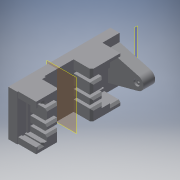
# Autodesk Inventor part: Assembly-jig-base
Saved by Autodesk Inventor 2018 (Build 220112000, 112)
## iProperties
Created: 2017-11-08
Part Number: Assembly-jig-base
Material: Generic
Document SubType Name: Modeling
Designer: xl0
Density: 1 g/cm^3
Appearance: Default
Author: xl0
Autodesk Inventor part; units mm, degrees
ref_plane "YZ Plane" through (0, 0, 0) normal (1, 0, 0) x (0, 1, 0)
ref_plane "XZ Plane" through (0, 0, 0) normal (0, 1, 0) x (-1, 0, 0)
ref_plane "Work Plane3" through (-2, 0, -40) normal (-1, 0, 0) x (0, 0, 1)
sketch "Sketch3" plane through (-2, 0, -8) normal (-1, 0, 0) x (0, -1, 0)
  line L0 (54.7526, 13.2) -> (67.7526, 13.2)
  line L1 (67.7526, 13.2) -> (67.7526, 3.2)
  line L2 (67.7526, 3.2) -> (54.7526, 3.2)
  line L3 (54.7526, 3.2) -> (54.7526, 13.2)
  line L4 (104.2526, 13.2) -> (117.2526, 13.2)
  line L5 (117.2526, 13.2) -> (117.2526, 3.2)
  line L6 (117.2526, 3.2) -> (104.2526, 3.2)
  line L7 (104.2526, 3.2) -> (104.2526, 13.2)
  line L8 (54.7526, -25.2) -> (67.7526, -25.2)
  line L9 (67.7526, -25.2) -> (67.7526, -35.2)
  line L10 (67.7526, -35.2) -> (54.7526, -35.2)
  line L11 (54.7526, -35.2) -> (54.7526, -25.2)
  line L12 (104.2526, -25.2) -> (117.2526, -25.2)
  line L13 (117.2526, -25.2) -> (117.2526, -35.2)
  line L14 (117.2526, -35.2) -> (104.2526, -35.2)
  line L15 (104.2526, -35.2) -> (104.2526, -25.2)
  line L16 (41.7526, -32) -> (41.7526, 8) projected
  line L17 (125.2526, 8) -> (125.2526, -32) projected
  line L18 (63.2526, 0) -> (63.2526, 3) projected
  line L19 (67.7526, 0) -> (67.7526, 3) projected
  line L20 (99.2526, 0) -> (99.2526, 3) projected
  line L21 (103.7526, 0) -> (103.7526, 3) projected
  line L22 (44.7526, 3) -> (122.2526, 3) projected
  line L23 (122.2526, -25) -> (44.7526, -25) projected
  line L24 (54.7526, -0.2) -> (67.7526, -0.2)
  line L25 (67.7526, -0.2) -> (67.7526, -11.8)
  line L26 (67.7526, -11.8) -> (54.7526, -11.8)
  line L27 (54.7526, -11.8) -> (54.7526, -0.2)
  line L28 (54.7526, -15.2) -> (67.7526, -15.2)
  line L29 (67.7526, -15.2) -> (67.7526, -21.8)
  line L30 (67.7526, -21.8) -> (54.7526, -21.8)
  line L31 (54.7526, -21.8) -> (54.7526, -15.2)
  line L32 (104.2526, -0.2) -> (117.2526, -0.2)
  line L33 (117.2526, -0.2) -> (117.2526, -11.8)
  line L34 (117.2526, -11.8) -> (104.2526, -11.8)
  line L35 (104.2526, -11.8) -> (104.2526, -0.2)
  line L36 (104.2526, -15.2) -> (117.2526, -15.2)
  line L37 (117.2526, -15.2) -> (117.2526, -21.8)
  line L38 (117.2526, -21.8) -> (104.2526, -21.8)
  line L39 (104.2526, -21.8) -> (104.2526, -15.2)
  line L40 (44.7526, 0) -> (122.2526, 0) projected
  line L41 (44.7526, -12) -> (122.2526, -12) projected
  line L42 (44.7526, -15) -> (122.2526, -15) projected
  line L43 (44.7526, -22) -> (122.2526, -22) projected
  line L44 (122.2526, 8) -> (122.2526, -32) projected
  line L45 (44.7526, -32) -> (44.7526, 8) projected
  line L46 (125.2526, 8) -> (122.2526, 8) projected
  line L47 (125.2526, -32) -> (122.2526, -32) projected
  dimension "d7" = 10
  dimension "d9" = 0.2
  dimension "d10" = 0.2
  dimension "d11" = 0.2
  dimension "d12" = 0.2
  dimension "d13" = 0.2
  dimension "d34" = 5
  dimension "d36" = 13
  dimension "d48" = 0.2
  dimension "d80" = 10
  constraints: 64 end point, 15 collinear, 15 parallel, 8 horizontal, 8 perpendicular, 4 equal length, 3 point on line
  measures "d7" distance of L0.end L1.end
  measures "d9" distance between parallel lines of L23 L8
  measures "d10" distance between parallel lines of L26 L41
  measures "d11" distance between parallel lines of L40 L24
  measures "d12" distance between parallel lines of L42 L28
  measures "d13" distance between parallel lines of L43 L30
  measures "d34" distance between parallel lines of L37 L44
  measures "d36" distance of L9.end L10.end
  measures "d48" distance between parallel lines of L22 L2
  measures "d80" distance between parallel lines of L11 L45
extrude "Extrusion2" add sketch "Sketch3" against normal blind 20 contours L0 L1 L2 L3 | L4 L5 L6 L7 | L8 L9 L10 L11 | L12 L13 L14 L15 | L24 L25 L26 L27 | L28 L29 L30 L31 | L32 L33 L34 L35 | L36 L37 L38 L39
sketch "Sketch10" plane through (-2, 0, -8) normal (-1, 0, 0) x (0, 0, 1)
  line L0 (13.2, -117.2526) -> (13.2, -129.2526)
  line L1 (13.2, -129.2526) -> (6.7, -129.2526)
  line L2 (6.7, -129.2526) -> (6.7, -125.4526)
  line L3 (6.7, -125.4526) -> (8.2, -125.4526)
  line L4 (6.7, -117.2526) -> (13.2, -117.2526)
  line L5 (8, -125.2526) -> (-32, -125.2526) projected
  line L6 (8, -125.2526) -> (8, -122.2526) projected
  line L7 (-32, -122.2526) -> (8, -122.2526) projected
  line L8 (-32, -125.2526) -> (-32, -122.2526) projected
  line L9 (13.2, -104.2526) -> (13.2, -117.2526) projected
  line L10 (-30.7, -129.2526) -> (-37.2, -129.2526)
  line L11 (-37.2, -129.2526) -> (-37.2, -104.2526)
  line L12 (-32.2, -125.4526) -> (-30.7, -125.4526)
  line L13 (-30.7, -125.4526) -> (-30.7, -129.2526)
  line L14 (-32.2, -125.4526) -> (-32.2, -122.0526)
  line L15 (-32.2, -122.0526) -> (-30.7, -122.0526)
  line L16 (-30.7, -122.0526) -> (-30.7, -117.2526)
  line L17 (8.2, -125.4526) -> (8.2, -122.0526)
  line L18 (8.2, -122.0526) -> (6.7, -122.0526)
  line L19 (6.7, -122.0526) -> (6.7, -117.2526)
  line L20 (13.2, -117.2526) -> (3.2, -117.2526) projected
  line L21 (-25.2, -104.2526) -> (-25.2, -117.2526) projected
  line L22 (-25.2, -117.2526) -> (-35.2, -117.2526) projected
  line L23 (-35.2, -117.2526) -> (-35.2, -104.2526) projected
  line L24 (-35.2, -104.2526) -> (-25.2, -104.2526) projected
  line L25 (-35.2, -117.2526) -> (-35.2, -104.2526) projected
  line L26 (-35.2, -104.2526) -> (-37.2, -104.2526)
  line L27 (13.2, -35.7526) -> (13.2, -54.7526)
  line L28 (5.2, -45.2526) -> (8.2, -45.2526)
  line L29 (8.2, -45.2526) -> (8.2, -35.7526)
  line L30 (8.2, -35.7526) -> (13.2, -35.7526)
  line L31 (-29.2, -45.2526) -> (-29.2, -54.7526)
  line L32 (-37.2, -67.7526) -> (-37.2, -35.7526)
  line L33 (-37.2, -35.7526) -> (-32.2, -35.7526)
  line L34 (-32.2, -35.7526) -> (-32.2, -45.2526)
  line L35 (-32.2, -45.2526) -> (-29.2, -45.2526)
  line L36 (8, -44.7526) -> (-32, -44.7526) projected
  line L37 (8, -44.7526) -> (8, -41.7526) projected
  line L38 (-32, -41.7526) -> (8, -41.7526) projected
  line L39 (-32, -44.7526) -> (-32, -41.7526) projected
  line L40 (13.2, -54.7526) -> (13.2, -67.7526) projected
  line L41 (13.2, -67.7526) -> (3.2, -67.7526) projected
  line L42 (3.2, -67.7526) -> (3.2, -54.7526) projected
  line L43 (3.2, -54.7526) -> (13.2, -54.7526) projected
  line L44 (3.2, -54.7526) -> (13.2, -54.7526) projected
  line L45 (-25.2, -54.7526) -> (-25.2, -67.7526) projected
  line L46 (-25.2, -67.7526) -> (-35.2, -67.7526) projected
  line L47 (-35.2, -67.7526) -> (-35.2, -54.7526) projected
  line L48 (-35.2, -54.7526) -> (-25.2, -54.7526) projected
  line L49 (-37.2, -67.7526) -> (-35.2, -67.7526)
  line L50 (5.2, -45.2526) -> (5.2, -54.7526)
  line L51 (-35.2, -54.7526) -> (-25.2, -54.7526) projected
  point P0 (8, 0)
  dimension "d50" = 0.2
  dimension "d54" = 12
  dimension "d58" = 0.2
  dimension "d59" = 0.2
  dimension "d60" = 1.5
  dimension "d61" = 0.2
  dimension "d71" = 0.5
  dimension "d72" = 0.2
  dimension "d75" = 6
  dimension "d77" = 5
  dimension "d78" = 0.2
  dimension "d79" = 0.5
  dimension "d83" = 3
  constraints: 54 end point, 12 collinear, 12 perpendicular, 5 horizontal, 4 point on line, 4 vertical, 3 parallel
  measures "d50" distance between parallel lines of L3 L5
  measures "d54" distance of L0.start L0.end
  measures "d58" distance between parallel lines of L17 L6
  measures "d59" distance between parallel lines of L18 L7
  measures "d60" distance of L17.end L18.end
  measures "d61" distance between parallel lines of L8 L14
  measures "d71" distance between parallel lines of L28 L36
  measures "d72" distance between parallel lines of L29 L37
  measures "d75" distance between parallel lines of L38 L30
  measures "d77" distance of L29.end L27.start
  measures "d78" distance between parallel lines of L39 L34
  measures "d79" distance between parallel lines of L35 L36
  measures "d83" distance of L28.start L28.end
extrude "Extrusion7" add sketch "Sketch10" against normal blind 20 contours L0 L1 L2 L3 L17 L18 L19 L4 | L10 L11 L26 L23 L22 L16 L15 L14 L12 L13 | L27 L43 L50 L28 L29 L30 | L31 L48 L47 L49 L32 L33 L34 L35
sketch "Sketch11" plane through (-2, 0, -8) normal (-1, 0, 0) x (0, 0, 1)
  line L0 (6.7, -122.0526) -> (6.7, -117.2526) projected
  line L1 (8.2, -122.0526) -> (6.7, -122.0526) projected
  line L2 (8.2, -125.4526) -> (8.2, -122.0526) projected
  line L3 (6.7, -125.4526) -> (8.2, -125.4526) projected
  line L4 (6.7, -129.2526) -> (6.7, -125.4526) projected
  line L5 (13.2, -129.2526) -> (6.7, -129.2526) projected
  line L6 (-37.2, -129.2526) -> (-30.7, -129.2526) projected
  line L7 (-30.7, -129.2526) -> (-30.7, -125.4526) projected
  line L8 (-30.7, -125.4526) -> (-32.2, -125.4526) projected
  line L9 (-32.2, -125.4526) -> (-32.2, -122.0526) projected
  line L10 (-32.2, -122.0526) -> (-30.7, -122.0526) projected
  line L11 (-30.7, -122.0526) -> (-30.7, -117.2526) projected
  line L12 (-37.2, -104.2526) -> (-37.2, -129.2526) projected
  line L13 (6.7, -122.0526) -> (6.7, -125.4526)
  line L14 (-30.7, -122.0526) -> (-32.2, -122.0526) projected
  line L15 (-30.7, -122.0526) -> (-30.7, -125.4526)
  line L16 (-11.8, -54.7526) -> (-0.2, -54.7526) projected
  line L17 (-25.2, -104.2526) -> (-25.2, -117.2526) projected
  line L18 (-25.2, -117.2526) -> (-30.7, -117.2526) projected
  line L19 (13.2, -104.2526) -> (13.2, -129.2526) projected
  line L20 (3.2, -104.2526) -> (13.2, -104.2526) projected
  line L21 (3.2, -117.2526) -> (3.2, -104.2526) projected
  line L22 (6.7, -117.2526) -> (3.2, -117.2526) projected
  line L23 (-25.2, -104.2526) -> (-37.2, -104.2526) projected
  line L24 (-25.2, -54.7526) -> (-25.2, -67.7526) projected
  line L25 (-29.2, -54.7526) -> (-25.2, -54.7526) projected
  line L26 (-29.2, -54.7526) -> (-29.2, -45.2526) projected
  line L27 (-29.2, -45.2526) -> (-32.2, -45.2526) projected
  line L28 (-32.2, -45.2526) -> (-32.2, -35.7526) projected
  line L29 (-32.2, -35.7526) -> (-37.2, -35.7526) projected
  line L30 (-37.2, -35.7526) -> (-37.2, -67.7526) projected
  line L31 (-25.2, -67.7526) -> (-37.2, -67.7526) projected
  line L32 (13.2, -35.7526) -> (13.2, -67.7526) projected
  line L33 (13.2, -35.7526) -> (8.2, -35.7526) projected
  line L34 (8.2, -35.7526) -> (8.2, -45.2526) projected
  line L35 (8.2, -45.2526) -> (5.2, -45.2526) projected
  line L36 (5.2, -45.2526) -> (5.2, -54.7526) projected
  line L37 (3.2, -54.7526) -> (5.2, -54.7526) projected
  line L38 (3.2, -67.7526) -> (3.2, -54.7526) projected
  line L39 (13.2, -67.7526) -> (3.2, -67.7526) projected
  line L40 (5.2, -45.2526) -> (5.2, -35.7526)
  line L41 (5.2, -35.7526) -> (8.2, -35.7526)
  line L42 (5.2, -45.2526) -> (5.2, -54.7526) projected
  line L43 (-29.2, -45.2526) -> (-29.2, -35.7526)
  line L44 (-29.2, -35.7526) -> (-32.2, -35.7526)
  line L45 (13.2, -35.7526) -> (8.2, -35.7526) projected
  point P0 (8, 0)
  constraints: 12 end point, 4 point on line, 3 perpendicular, 2 collinear, 2 vertical, 1 parallel
ref_plane "Work Plane5" through (0, -122.2526, -8) normal (-1, 0, 0) x (0, 0, 1)
extrude "Extrusion8" add sketch "Sketch11" against normal up to surface (2 mm away) contours L1 L2 L3 L13 | L12 L23 L17 L18 L11 L10 L9 L8 L7 L6 | L27 L28 L44 L43 | L32 L39 L38 L37 L36 L35 L34 L33
sketch "Sketch4" plane through (-2, 0, -8) normal (-1, 0, 0) x (0, 0, 1)
  line L0 (13.2, -16.7526) -> (-37.2, -16.7526)
  line L1 (-37.2, -16.7526) -> (-37.2, -130.2526)
  line L2 (-37.2, -130.2526) -> (13.2, -130.2526)
  line L3 (13.2, -130.2526) -> (13.2, -16.7526)
  line L4 (13.2, -35.7526) -> (13.2, -67.7526) projected
  line L5 (3.2, -67.7526) -> (3.2, -54.7526) projected
  line L6 (13.2, -67.7526) -> (3.2, -67.7526) projected
  line L7 (13.2, -104.2526) -> (13.2, -129.2526) projected
  line L8 (3.2, -104.2526) -> (13.2, -104.2526) projected
  line L9 (3.2, -117.2526) -> (3.2, -104.2526) projected
  line L10 (6.7, -117.2526) -> (3.2, -117.2526) projected
  line L11 (-25.2, -54.7526) -> (-25.2, -67.7526) projected
  line L12 (-29.2, -54.7526) -> (-25.2, -54.7526) projected
  line L13 (-25.2, -67.7526) -> (-37.2, -67.7526) projected
  line L14 (-25.2, -104.2526) -> (-25.2, -117.2526) projected
  line L15 (-25.2, -104.2526) -> (-37.2, -104.2526) projected
  line L16 (-25.2, -117.2526) -> (-30.7, -117.2526) projected
  line L17 (-32, -41.7526) -> (8, -41.7526) projected
  line L18 (8, -125.2526) -> (-32, -125.2526) projected
  line L19 (13.2, -54.7526) -> (13.2, -67.7526) projected
  line L20 (-35.2, -67.7526) -> (-35.2, -54.7526) projected
  line L21 (6.7, -129.2526) -> (6.7, -117.2526) projected
  line L22 (13.2, -129.2526) -> (6.7, -129.2526) projected
  line L23 (-37.2, -104.2526) -> (-37.2, -129.2526) projected
  line L24 (-37.2, -129.2526) -> (-30.7, -129.2526) projected
  line L25 (-30.7, -129.2526) -> (-30.7, -125.4526) projected
  line L26 (-30.7, -125.4526) -> (-32.2, -125.4526) projected
  line L27 (-32.2, -125.4526) -> (-32.2, -122.0526) projected
  line L28 (-32.2, -122.0526) -> (-30.7, -122.0526) projected
  line L29 (-30.7, -122.0526) -> (-30.7, -117.2526) projected
  line L30 (-37.2, -129.2526) -> (-37.2, -104.2526) projected
  line L31 (-37.2, -35.7526) -> (-37.2, -67.7526) projected
  line L32 (13.2, -35.7526) -> (8.2, -35.7526) projected
  line L33 (5.2, -45.2526) -> (5.2, -54.7526) projected
  line L34 (3.2, -54.7526) -> (5.2, -54.7526) projected
  line L35 (-29.2, -54.7526) -> (-29.2, -35.7526) projected
  line L36 (-29.2, -35.7526) -> (-37.2, -35.7526) projected
  line L37 (8.2, -35.7526) -> (8.2, -45.2526) projected
  line L38 (8.2, -45.2526) -> (5.2, -45.2526) projected
  point P0 (8, 0)
  dimension "d16" = 25
  dimension "d17" = 5
  constraints: 8 end point, 2 collinear, 2 parallel, 1 horizontal, 1 perpendicular
  measures "d16" distance between parallel lines of L0 L17
  measures "d17" distance between parallel lines of L2 L18
extrude "Extrusion3" add sketch "Sketch4" along normal blind 10
sketch "Sketch6" plane through (-2, -16.7526, 5.2) normal (0, 1, 0) x (1, 0, 0)
  arc A0 (33.9411, 17.9556) -> (33.9411, 32.4444) centre (32, 25.2) ccw
  line L0 (0, 0) -> (0, 50.4) projected
  line L1 (33.9411, 32.4444) -> (0, 41.5389)
  line L2 (0, 28.4) -> (0, 35) projected
  line L3 (33.9411, 17.9556) -> (0, 8.8611)
  line L4 (0, 50.4) -> (0, 0) projected
  point P0 (2, 5.2)
  point P1 (0, 25.2)
  dimension "d21" = 15
  dimension "d22" = 75
  dimension "d23" = 75
  dimension "d68" = 32
  constraints: 4 end point, 2 point on circle, 2 point on line, 2 tangent, 1 centre point, 1 horizontal alignment, 1 midpoint
  measures "d21" diameter of A0
  measures "d22" angle of L4 L1
  measures "d23" angle of L0 L3
  measures "d68" distance from line of L0 A0.centre
extrude "Extrusion4" add sketch "Sketch6" against normal blind 13
sketch "Sketch7" plane through (-2, -29.7526, 5.2) normal (0, -1, 0) x (1, 0, 0)
  arc A0 (33.9411, -32.4444) -> (33.9411, -17.9556) centre (32, -25.2) ccw projected
  line L0 (0, -8.8611) -> (33.9411, -17.9556) projected
  line L1 (33.9411, -32.4444) -> (0, -41.5389) projected
  point P0 (2, -5.2)
hole "Hole1" at (30, -29.7526, -20) direction (0, 1, 0) diameter 3 end through all counterbore diameter 7 counterbore depth 2
ref_plane "Work Plane4" through (18, -86.0026, -4.8) normal (0, -1, 0) x (1, 0, 0)
sketch "Sketch8" plane through (18, -67.7526, 5.2) normal (0, 0, 1) x (1, 0, 0)
  line L0 (-20, 51) -> (-20, -62.5) projected
  line L1 (-20, 18) -> (-18.5, 18)
  line L2 (-18.5, 18) -> (-18.5, 8)
  line L3 (-18.5, 8) -> (-20, 8)
  line L4 (-20, 0) -> (0, 0) projected
  line L5 (-20, 0) -> (-9.8118, 0) construction
  line L6 (-20, -49.5) -> (-20, -36.5) projected
  line L7 (-20, -32.3) -> (-18.5, -32.3)
  line L8 (-18.5, -52.3) -> (-18.5, -32.3)
  line L9 (-18.5, -52.3) -> (-20, -52.3)
  line L10 (-20, -61.5) -> (-20, -49.5) projected
  line L11 (-18, -54.3) -> (0, -54.3) projected
  line L12 (-20, -36.5) -> (-20, 0) projected
  line L13 (41.5, 23) -> (-18, 23) projected
  point P0 (-18, 67.7526)
  point P1 (-20, -59.3)
  dimension "d38" = 1.5
  dimension "d39" = 10
  dimension "d69" = 2
  dimension "d70" = 20
  dimension "d82" = 5
  constraints: 14 end point, 5 perpendicular, 5 point on line, 1 collinear, 1 horizontal, 1 other
  measures "d38" distance between parallel lines of L0 L2
  measures "d39" distance between parallel lines of L3 L1
  measures "d70" distance of L8.start L7.end
  measures "d82" distance between parallel lines of L1 L13
extrude "Extrusion5" add sketch "Sketch8" against normal up to surface (50.4 mm away)
chamfer "Chamfer1" distance 2 angle 45 34 edges at (18, -61.2526, -33.2) (18, -61.2526, -29.8) (18, -61.2526, -19.8) (18, -61.2526, -8.2) (18, -61.2526, -4.8) (18, -67.7526, 0.2) (18, -67.7526, -14) (18, -67.7526, -26.5) (18, -67.7526, -39.2) (18, -61.2526, -23.2) (18, -54.7526, -35.2) (18, -54.7526, -26.5) (18, -54.7526, -14) (18, -54.7526, -3.8) (18, -104.2526, -39.2) (18, -104.2526, -26.5) (18, -104.2526, -14) (18, -104.2526, 0.2) (18, -110.7526, -4.8) (18, -110.7526, -8.2) (18, -110.7526, -19.8) (18, -110.7526, -23.2) (18, -110.7526, -29.8) (18, -110.7526, -33.2) (18, -122.0526, -39.45) (18, -123.7526, -40.2) (18, -125.4526, -39.45) (18, -123.7526, 0.2) (18, -122.0526, -0.55) (18, -125.4526, -0.55) (18, -40.5026, 0.2) (18, -45.2526, -1.3) (18, -45.2526, -38.7) (18, -40.5026, -40.2)
equation "\"d10\" = d9"
equation "\"d11\" = d9"
equation "\"d12\" = d9"
equation "\"d13\" = d9"
equation "\"d48\" = d9"
equation "\"d58\" = d50"
equation "\"d59\" = d50"
equation "\"d61\" = d50"
body "Solid2"
